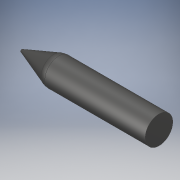
# Autodesk Inventor part: elekrode_tip_t
Saved by Autodesk Inventor 2017 (Build 210142000, 142)
## iProperties
Part Number: elekrode_tip_t
Material: Generisch
Document SubType Name: Modeling
Designer: David Merges
Density: 1 g/cm^3
Appearance: Wolfram
Author: David Merges
Autodesk Inventor part; units mm, degrees
ref_plane "YZ Plane" through (0, 0, 0) normal (1, 0, 0) x (0, 1, 0)
ref_plane "XZ Plane" through (0, 0, 0) normal (0, 1, 0) x (-1, 0, 0)
ref_plane "XY Plane" through (0, 0, 0) normal (0, 0, 1) x (1, 0, 0)
sketch "Skizze1" plane through (0, 0, 0) normal (1, 0, 0) x (0, 1, 0)
  circle A0 centre (0, 0) radius 0.5
  dimension "d0" = 1
  constraints: 1 centre point, 1 coincident
  measures "d0" diameter of A0
extrude "Extrusion1" add sketch "Skizze1" along normal blind 5
sketch "Skizze2" plane through (0, 0, 0) normal (0, 0, 1) x (1, 0, 0)
  line L0 (5, -0.5) -> (5, 0.5) projected
  line L1 (0, 0.5) -> (0, -0.5) construction
  line L2 (0, 0.5) -> (5, 0.5) construction
  line L3 (0, 0.5) -> (0, -0.5) projected
  line L4 (0, 0) -> (0, 0.5)
  line L5 (0, 0.5) -> (1.2775, 0.5)
  line L6 (-1.1243, 0) -> (6.0207, 0) projected
  line L7 (1.2775, 0.5) -> (0.0329, 0.047)
  arc A0 (0.0329, 0.047) -> (0, 0) centre (0.05, 0) ccw
  dimension "d6" = 20
  dimension "d8" = 0.05
  constraints: 6 end point, 2 point on circle, 2 tangent, 1 centre point, 1 collinear, 1 perpendicular
  measures "d6" angle of L6 L7
  measures "d8" radius of A0
revolve "Umdrehung1" cut sketch "Skizze2" angle 360 about axis through (-10, 0, 0) along (1, 0, 0)
fillet "Rundung1" radius 0.5 1 edges at (1.2775, -0.5, 0)
